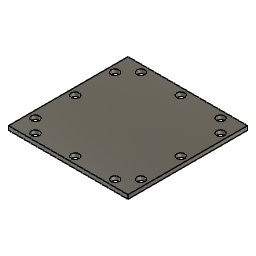
Basket Bottom v0 (1) (Autodesk Fusion 360 design; units mm, degrees)
Autodesk Fusion 360 part; units mm, degrees
sketch "Sketch1" plane through (0, 0, 0) normal (0, 0, 1) x (1, 0, 0)
  line L0 (0, 0) -> (60, 0)
  line L1 (60, 0) -> (60, -60)
  line L2 (60, -60) -> (0, -60)
  line L3 (0, -60) -> (0, 0)
  dimension "d1" = 60
  dimension "d2" = 60
  constraint horizontal L0
  constraint vertical L1
  constraint horizontal L2
  constraint vertical L3
  constraint coincident L0.start L3.end
  measures "d1" distance of L0.start L0.end
  measures "d2" distance of L0.start L2.end
extrude "Extrude1" add sketch "Sketch1" along normal blind 2
sketch "Sketch2" plane through (0, 0, 2) normal (0, 0, 1) x (-1, 0, 0)
  line L0 (0, 60) -> (-60, 60)
  line L1 (-60, 60) -> (-60, 0)
  line L2 (-60, 0) -> (0, 0)
  line L3 (0, 0) -> (0, 60)
  line L4 (-60, 10) -> (-56.5, 10)
  line L5 (-60, 3.5) -> (-50, 3.5)
  line L6 (-30, 0) -> (-30, 60)
  line L7 (0, 30) -> (-60, 30)
  line L8 (-30, 0) -> (-30, 3.5)
  line L9 (0, 30) -> (-3.5, 30)
  line L10 (-60, 30) -> (-56.5, 30)
  point P0 (-10, 3.5)
  point P1 (-3.5, 10)
  point P2 (-3.5, 50)
  point P3 (-10, 56.5)
  point P4 (-50, 56.5)
  point P5 (-56.5, 50)
  point P6 (-30, 56.5)
  dimension "d5" = 3.5
  dimension "d6" = 10
  dimension "d7" = 10
  dimension "d8" = 3.5
  dimension "d9" = 3.5
  dimension "d10" = 3.5
  dimension "d11" = 3.5
  constraint coincident L1 L4.start
  constraint perpendicular L1 L4
  constraint coincident L1 L5.start
  constraint perpendicular L1 L5
  constraint midpoint L2 L6.start
  constraint midpoint L0 L6.end
  constraint symmetric L4.end L6 P1
  constraint symmetric L5.end L6 P0
  constraint midpoint L3 L7.start
  constraint midpoint L1 L7.end
  constraint symmetric L4.end L7 P5
  constraint symmetric L5.end L7 P4
  constraint symmetric P0 L7 P3
  constraint symmetric P1 L7 P2
  constraint perpendicular L2 L8
  constraint symmetric L7 L8.end P6
  constraint perpendicular L3 L9
  constraint perpendicular L1 L10
  measures "d5" distance of L4.start L4.end
  measures "d6" distance of L2 L4.end
  measures "d7" distance of L5.start L5.end
  measures "d8" distance of L2 L5
  measures "d9" distance of L6.start L8.end
  measures "d10" distance of L7.start L9.end
  measures "d11" distance of L7.end L10.end
hole "Hole1" at (10, -3.5, 2) at (3.5, -10, 2) at (3.5, -30, 2) at (3.5, -50, 2) at (10, -56.5, 2) at (30, -56.5, 2) at (50, -56.5, 2) at (56.5, -50, 2) at (56.5, -30, 2) at (56.5, -10, 2) at (50, -3.5, 2) at (30, -3.5, 2) direction (0, 0, -1) diameter 4 depth 50 tip angle 180
